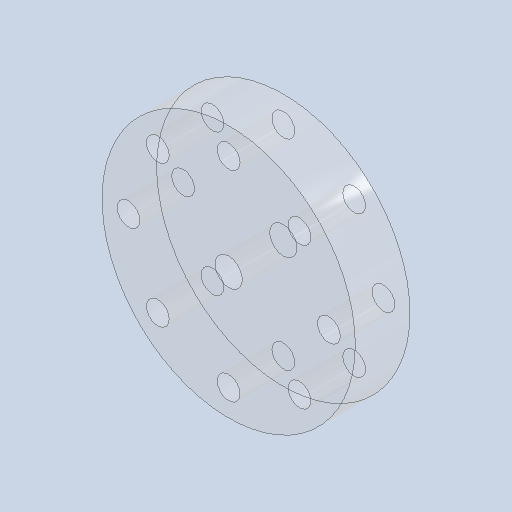
# Autodesk Inventor part: _idle-pelvis_adt
Saved by Autodesk Inventor 2024.3 (Build 283343000, 343)
## iProperties
Created: 2024-09-08
Part Number: _idle-pelvis_adt
Material: PMMA 플라스틱
Document SubType Name: Modeling
Designer: gretc
Density: 1.188 g/cm^3
Appearance: 폴리카보네이트 - 선명
Mass: 3.9963 g
Surface Area: 20.7885 cm^2
Volume: 3.36389 cm^3
Author: gretc
Autodesk Inventor part; units mm, degrees
ref_plane "YZ Plane" through (0, 0, 0) normal (1, 0, 0) x (0, 1, 0)
ref_plane "XZ Plane" through (0, 0, 0) normal (0, 1, 0) x (-1, 0, 0)
ref_plane "XY Plane" through (0, 0, 0) normal (0, 0, 1) x (1, 0, 0)
sketch "스케치1" plane through (0, 0, 0) normal (0, 0, 1) x (1, 0, 0)
  circle A0 centre (-11, 0) radius 1.25 projected
  circle A1 centre (11, 0) radius 1.25 projected
  circle A2 centre (7.7782, -7.7782) radius 1.25 projected
  circle A3 centre (-7.7782, 7.7782) radius 1.25 projected
  circle A4 centre (-7.7782, -7.7782) radius 1.25 projected
  circle A5 centre (7.7782, 7.7782) radius 1.25 projected
  circle A6 centre (0, -11) radius 1.25 projected
  circle A7 centre (0, 11) radius 1.25 projected
  circle A8 centre (0, 0) radius 1.5 projected
  circle A9 centre (0, 0) radius 13.9 projected
  point P0 (0, 0)
extrude "돌출1" add sketch "스케치1" along normal blind 6
